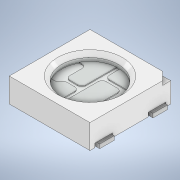
# Autodesk Inventor part: WS2812b_SMD
Saved by Autodesk Inventor 2020 (Build 240168000, 168)
## iProperties
Created: 2020-03-29
Part Number: WS2812b_SMD
Material: Generic
Document SubType Name: Modeling
Designer: ermoz
Density: 1 g/cm^3
Appearance: Default
Author: ermoz
Autodesk Inventor part; units mm, degrees
ref_plane "YZ Plane" through (0, 0, 0) normal (1, 0, 0) x (0, 1, 0)
ref_plane "XZ Plane" through (0, 0, 0) normal (0, 1, 0) x (-1, 0, 0)
ref_plane "XY Plane" through (0, 0, 0) normal (0, 0, 1) x (1, 0, 0)
sketch "Sketch1" plane through (0, 0, 0) normal (0, 1, 0) x (-1, 0, 0)
  line L0 (-2.5, 2.5) -> (2.5, 2.5)
  line L1 (2.5, 2.5) -> (2.5, -2.5)
  line L2 (2.5, -2.5) -> (-2.5, -2.5)
  line L3 (-2.5, -2.5) -> (-2.5, 2.5)
  line L4 (-2.5, 2.5) -> (2.5, -2.5) construction
  line L5 (2.5, 2.5) -> (-2.5, -2.5) construction
  point P0 (0, 0)
  dimension "d0" = 5
  dimension "d1" = 5
  constraints: 12 end point, 2 midpoint, 2 parallel, 1 horizontal, 1 perpendicular
  measures "d0" distance of L1.end L2.end
  measures "d1" distance of L0.end L1.end
extrude "Extrusion1" add sketch "Sketch1" along normal blind 1
sketch "Sketch2" plane through (0, 1, 0) normal (0, 1, 0) x (1, 0, 0)
  circle A0 centre (0, 0) radius 2
  circle A1 centre (0, 0) radius 1.75
  dimension "d4" = 4
  dimension "d5" = 3.5
  constraints: 2 centre point, 2 coincident
  measures "d4" diameter of A0
  measures "d5" diameter of A1
extrude "Extrusion2" add sketch "Sketch2" along normal blind 0.25
sketch "Sketch3" plane through (0, 1, 0) normal (0, 1, 0) x (1, 0, 0)
  line L0 (0.1, -2.6193) -> (-0.1, -2.6193)
  line L1 (-0.1, -2.6193) -> (-0.1, -0.85)
  line L2 (-0.1, 2.6193) -> (0.1, 2.6193)
  line L3 (0.1, 0.4) -> (0.1, -2.6193)
  line L4 (0, 0) -> (0, -0.5)
  line L5 (-0.35, -0.6) -> (-0.85, -0.6)
  line L6 (-2.9966, -0.6) -> (-2.9966, -0.4)
  line L7 (-0.85, -0.4) -> (-0.35, -0.4)
  line L8 (2.9966, -0.4) -> (2.9966, -0.6)
  line L9 (0, 0) -> (0, 0.5)
  line L10 (0, 0.5) -> (0, 0.75)
  line L11 (1.05, 0.65) -> (0.35, 0.65)
  line L12 (-3.251, 0.65) -> (-3.251, 0.85)
  line L13 (-3.251, 0.85) -> (-1.35, 0.85)
  line L14 (3.251, 0.85) -> (3.251, 0.65)
  line L15 (0, 0.75) -> (1.4, 0.75)
  line L16 (0, -0.5) -> (-1.2, -0.5)
  line L17 (-1.3, -2.7729) -> (-1.1, -2.7729)
  line L18 (-1.1, -2.7729) -> (-1.1, -0.85)
  line L19 (-1.1, 1.7729) -> (-1.3, 1.7729)
  line L20 (-1.3, 1.7729) -> (-1.3, -2.7729)
  line L21 (1.3, 3.2834) -> (1.5, 3.2834)
  line L22 (1.5, 3.2834) -> (1.5, -1.7834)
  line L23 (1.5, -1.7834) -> (1.3, -1.7834)
  line L24 (1.3, -0.6514) -> (1.3, 0.4)
  line L25 (1.3, 3.2834) -> (1.5, -1.7834) construction
  line L26 (1.5, 3.2834) -> (1.3, -1.7834) construction
  circle A0 centre (0, 0) radius 1.75
  circle A1 centre (0, 0) radius 1.75 projected
  line L27 (1.5, -0.9014) -> (1.55, -0.9014)
  arc A2 (1.3, -0.6514) -> (1.55, -0.9014) centre (1.55, -0.6514) ccw
  arc A3 (1.3, 0.4) -> (1.05, 0.65) centre (1.05, 0.4) ccw
  arc A4 (0.35, 0.65) -> (0.1, 0.4) centre (0.35, 0.4) ccw
  arc A5 (-0.1, -0.85) -> (-0.35, -0.6) centre (-0.35, -0.85) ccw
  arc A6 (-0.85, -0.6) -> (-1.0794, -0.7507) centre (-0.85, -0.85) ccw
  line L28 (-1.3089, -0.9014) -> (-1.5, -0.9014)
  arc A7 (-1.3089, -0.9014) -> (-1.0794, -0.7507) centre (-1.3089, -0.6514) ccw
  line L29 (-1.1, -0.15) -> (-1.1, 0.6)
  line L30 (3.251, 0.65) -> (-3.251, 0.65)
  line L31 (-0.1, 2.6193) -> (-0.1, -0.15)
  arc A8 (-0.35, -0.4) -> (-0.1, -0.15) centre (-0.35, -0.15) ccw
  arc A9 (-1.1, -0.15) -> (-0.85, -0.4) centre (-0.85, -0.15) ccw
  arc A10 (-1.1, 0.6) -> (-1.35, 0.85) centre (-1.35, 0.6) ccw
  line L32 (0.1, 1.1) -> (0.1, 2.0881)
  line L33 (0.35, 0.85) -> (3.251, 0.85)
  arc A11 (0.1, 1.1) -> (0.35, 0.85) centre (0.35, 1.1) ccw
  point P0 (0.1, -1.7471)
  point P1 (1.5, -0.9014)
  point P2 (1.5, -0.8963)
  point P3 (-0.1, -1.7471)
  point P4 (1.5297, 0.85)
  point P5 (0.1, 1.7471)
  point P6 (-0.1, 1.7471)
  point P7 (-1.5297, 0.85)
  dimension "d8" = 0.2
  dimension "d9" = 0.5
  dimension "d10" = 0.2
  dimension "d11" = 0.5
  dimension "d12" = 0.25
  dimension "d13" = 0.2
  dimension "d14" = 1.4
  dimension "d15" = 1.2
  dimension "d16" = 0.2
  dimension "d17" = 0.2
  dimension "d18" = 0.25
  dimension "d19" = 0.25
  dimension "d20" = 0.25
  dimension "d21" = 0.25
  constraints: 68 end point, 23 point on circle, 21 tangent, 20 point on line, 12 parallel, 11 centre point, 8 perpendicular, 6 equal radius, 6 horizontal, 5 vertical, 2 midpoint, 1 coincident, 1 collinear
  measures "d8" distance of L2.start L2.end
  measures "d9" distance of L4.start L4.end
  measures "d10" distance of L6.start L6.end
  measures "d11" distance of L4.start L9.end
  measures "d12" distance of L9.end L10.end
  measures "d13" distance of L12.start L12.end
  measures "d14" distance of L10.end L15.end
  measures "d15" distance of L4.end L16.end
  measures "d16" distance of L19.end L19.start
  measures "d17" distance of L22.end L23.end
  measures "d18" radius of A2
  measures "d19" radius of A7
  measures "d20" radius of A8
  measures "d21" radius of A11
extrude "Extrusion3" add sketch "Sketch3" along normal blind 0.05 separate body contours L3 A4 L11 A3 L24 A2 A0 | A0 L20 A7 A6 L5 A5 L1 | A0 L28 A7 L20 | L33 A11 L32 A0 L22 | L22 A0 L33 | L31 A8 L7 A9 L29 A10 L30 | L30 A10 L20 A0 L31 | A10 L13 A0 L20
sketch "Sketch4" plane through (0, 0, 0) normal (0, -1, 0) x (1, 0, 0)
  line L0 (2.7, 2.1) -> (-2.7, 2.1)
  line L1 (-2.7, 2.1) -> (-2.7, -2.1)
  line L2 (-2.7, -2.1) -> (2.7, -2.1)
  line L3 (2.7, -2.1) -> (2.7, 2.1)
  line L4 (2.7, 2.1) -> (-2.7, -2.1) construction
  line L5 (-2.7, 2.1) -> (2.7, -2.1) construction
  line L6 (2.7, -2.1) -> (1.8, -2.1)
  line L7 (1.8, -2.1) -> (1.8, -1.2)
  line L8 (1.8, -1.2) -> (2.7, -1.2)
  line L9 (2.7, -1.2) -> (2.7, -2.1)
  line L10 (2.7, 2.1) -> (1.8, 2.1)
  line L11 (1.8, 2.1) -> (1.8, 1.2)
  line L12 (1.8, 1.2) -> (2.7, 1.2)
  line L13 (2.7, 1.2) -> (2.7, 2.1)
  line L14 (-2.7, 2.1) -> (-1.8, 2.1)
  line L15 (-1.8, 2.1) -> (-1.8, 1.2)
  line L16 (-1.8, 1.2) -> (-2.7, 1.2)
  line L17 (-2.7, 1.2) -> (-2.7, 2.1)
  line L18 (-2.7, -2.1) -> (-1.8, -2.1)
  line L19 (-1.8, -2.1) -> (-1.8, -1.2)
  line L20 (-1.8, -1.2) -> (-2.7, -1.2)
  line L21 (-2.7, -1.2) -> (-2.7, -2.1)
  line L22 (1.7, -1.1) -> (1.7, -2.2)
  line L23 (1.7, -2.2) -> (2.8, -2.2)
  line L24 (2.8, -2.2) -> (2.8, -1.1)
  line L25 (2.8, -1.1) -> (1.7, -1.1)
  line L26 (1.7, 1.1) -> (1.7, 2.2)
  line L27 (1.7, 2.2) -> (2.8, 2.2)
  line L28 (2.8, 2.2) -> (2.8, 1.1)
  line L29 (2.8, 1.1) -> (1.7, 1.1)
  line L30 (-1.7, 1.1) -> (-1.7, 2.2)
  line L31 (-1.7, 2.2) -> (-2.8, 2.2)
  line L32 (-2.8, 2.2) -> (-2.8, 1.1)
  line L33 (-2.8, 1.1) -> (-1.7, 1.1)
  line L34 (-2.8, -1.1) -> (-1.7, -1.1)
  line L35 (-1.7, -1.1) -> (-1.7, -2.2)
  line L36 (-1.7, -2.2) -> (-2.8, -2.2)
  line L37 (-2.8, -2.2) -> (-2.8, -1.1)
  point P0 (0, 0)
  dimension "d24" = 5.4
  dimension "d25" = 4.2
  dimension "d26" = 0.9
  dimension "d27" = 0.9
  dimension "d28" = 0.9
  dimension "d29" = 0.9
  dimension "d30" = 0.9
  dimension "d31" = 0.9
  dimension "d32" = 0.9
  dimension "d33" = 0.9
  dimension "d34" = 0.1
  dimension "d35" = 0.1
  dimension "d36" = 0.1
  dimension "d37" = 0.1
  constraints: 76 end point, 18 parallel, 9 perpendicular, 5 horizontal, 2 midpoint, 12 other
  measures "d24" distance of L2.end L1.end
  measures "d25" distance of L1.end L0.end
  measures "d26" distance of L7.end L8.end
  measures "d27" distance of L6.end L7.end
  measures "d28" distance of L12.end L11.end
  measures "d29" distance of L11.end L10.end
  measures "d30" distance of L15.end L16.end
  measures "d31" distance of L14.end L15.end
  measures "d32" distance of L20.end L19.end
  measures "d33" distance of L19.end L18.end
  measures "d34" distance between parallel lines of L7 L22
  measures "d35" distance between parallel lines of L11 L26
  measures "d36" distance between parallel lines of L15 L30
  measures "d37" distance between parallel lines of L20 L34
extrude "Extrusion4" cut sketch "Sketch4" against normal blind 0.25 contours L3 L12 L11 L0 | L0 L26 L27 L28 L29 L3 | L11 L12 L3 L29 L26 L0 | L30 L33 L1 L16 L15 L0 | L0 L1 L33 L32 L31 L30 | L25 L24 L23 L22 L2 L3 | L3 L8 L7 L2 L22 L25 | L15 L16 L1 L0 | L3 L2 L7 L8 | L34 L35 L2 L19 L20 L1 | L1 L2 L35 L36 L37 L34 | L20 L19 L2 L1 bodies 1
extrude "Extrusion5" add sketch "Sketch4" against normal blind 0.25 separate body contours L3 L12 L11 L0 | L15 L16 L1 L0 | L3 L2 L7 L8 | L20 L19 L2 L1
sketch "Sketch5" plane through (0, 1, 0) normal (0, 1, 0) x (1, 0, 0)
  line L0 (-2.5, -2.5) -> (2.5, -2.5) projected
  line L1 (2.5, 2.5) -> (-2.5, 2.5) projected
  line L2 (-2.5, -2.5) -> (2.5, -2.5)
  line L3 (2.5, -2.5) -> (2.5, 2.5)
  line L4 (2.5, 2.5) -> (-2.5, 2.5)
  line L5 (-2.5, 2.5) -> (-2.5, -2.5)
  circle A0 centre (0, 0) radius 1.75
  constraints: 8 end point, 2 parallel, 1 centre point, 1 coincident, 1 horizontal, 1 perpendicular
extrude "Extrusion6" add sketch "Sketch5" along normal blind 0.5 bodies 1
sketch "Sketch6" plane through (0, 1.5, 0) normal (0, 1, 0) x (1, 0, 0)
  line L0 (2.5, 2.5) -> (-2.5, 2.5) projected
  line L1 (2.5, 2.5) -> (2, 2.5)
  line L2 (2, 2.5) -> (2.5, 2)
  line L3 (2.5, 1.1) -> (2.5, 2.2) projected
  line L4 (2.5, -2.5) -> (2.5, 2.5) projected
  line L5 (2.5, 2) -> (2.5, 2.5)
  point P0 (0, 0)
  dimension "d44" = 0.5
  dimension "d45" = 45
  constraints: 6 end point, 2 point on line, 1 collinear
  measures "d44" distance of L0.start L1.end
  measures "d45" angle of L2 L1
extrude "Extrusion7" cut sketch "Sketch6" against normal blind 0.25 bodies 1
chamfer "Chamfer1" distance 0.25 angle 45 1 edges at (-1.75, 1.5, 0)
sketch "Sketch7" plane through (0, 1.05, 0) normal (0, 1, 0) x (1, 0, 0)
  circle A0 centre (0, 0) radius 1.75
  constraints: 1 centre point, 1 coincident
extrude "Extrusion8" add sketch "Sketch7" along normal blind 0.2 separate body
body "Solid1"
body "Solid2"
body "Solid3"
body "Solid4"
